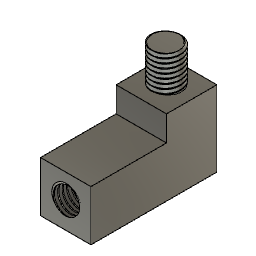
90block v4 (Autodesk Fusion 360 design; units mm, degrees)
Autodesk Fusion 360 part; units mm, degrees
box "BoxPrimitive1" add length 30 width 20 height 20 placed x (0, -1, 0) y (1, 0, 0) z (0, 0, 1) at (-20, 0, 0)
box "BoxPrimitive2" add length 20 width 30 height 20 placed x (0, 1, 0) y (-1, 0, 0) z (0, 0, 1) at (10, 0, 0)
cylinder "CylinderPrimitive1" add diameter 12 height 15 placed x (0, 0, -1) y (0, 1, 0) z (1, 0, 0) at (10, 10, 10)
cylinder "CylinderPrimitive2" cut diameter 12 height -15 placed x (1, 0, 0) y (0, 0, 1) z (0, -1, 0) at (-10, -30, 10)
thread "Thread2" "ISO Metric profile 12.0 M12x1.75 6H" major diameter 12.2265 minor diameter 10.2735 pitch 1.75 angle 60 modelled right hand crest width 0.4769 on face at (-4.0298, -20, 9.4026) crest through (-10, -29.5625, 15.1368)
thread "Thread4" "ISO Metric profile 12.0 M12x1.75 6g" major diameter 11.8335 minor diameter 9.8365 pitch 1.75 angle 60 modelled right hand crest width 0.2518 on face at (15, 9.4026, 4.0298) crest through (9.5625, 10, 4.0833)
move_body "Move1" bodies 1 to x (0, 0, 1) y (0, 1, 0) z (-1, 0, 0) at (-5, 0, 5)
